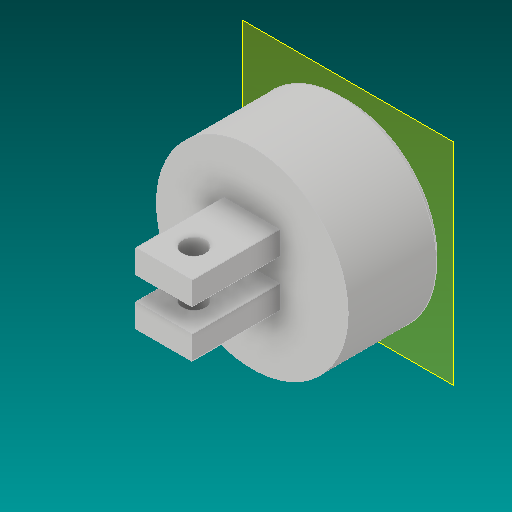
# Autodesk Inventor part: Swing_Joint_2
Saved by Autodesk Inventor 2019 (Build 230136000, 136)
## iProperties
Created: 2020-12-14
Part Number: Swing_Joint_2
Material: Generic
Document SubType Name: Modeling
Designer: Jason
Density: 1 g/cm^3
Appearance: Default
Mass: 7.35511 g
Surface Area: 26.6726 cm^2
Volume: 7.35511 cm^3
Author: Jason
Autodesk Inventor part; units mm, degrees
ref_plane "YZ Plane" through (0, 0, 0) normal (1, 0, 0) x (0, 1, 0)
ref_plane "XZ Plane" through (0, 0, 0) normal (0, 1, 0) x (-1, 0, 0)
ref_plane "XY Plane" through (0, 0, 0) normal (0, 0, 1) x (1, 0, 0)
ref_plane "Work Plane1" through (-10.8248, 8.3603, 0) normal (0, 0, 1) x (1, 0, 0)
sketch "Sketch3" plane through (-10.8248, 8.3603, 0) normal (0, 0, 1) x (1, 0, 0)
  circle A0 centre (0, 0) radius 12
  point P0 (0, 0)
  dimension "d0" = 24
  constraints: 1 centre point, 1 coincident
  measures "d0" diameter of A0
extrude "Extrusion1" add sketch "Sketch3" along normal blind 1
sketch "Sketch4" plane through (-10.8248, 8.3603, 1) normal (0, 0, 1) x (1, 0, 0)
  circle A0 centre (0, 0) radius 13
  circle A1 centre (0, 0) radius 12 projected
  dimension "d4" = 26
  constraints: 2 coincident, 1 centre point
  measures "d4" diameter of A0
extrude "Extrusion2" add sketch "Sketch4" along normal blind 12 contours A0 | A1
sketch "Sketch5" plane through (-10.8248, 8.3603, 13) normal (0, 0, 1) x (1, 0, 0)
  line L0 (-3.81, 2.1338) -> (3.81, 2.1338)
  line L1 (3.81, 2.1338) -> (3.81, 5.3088)
  line L2 (3.81, 5.3088) -> (-3.81, 5.3088)
  line L3 (-3.81, 5.3088) -> (-3.81, 2.1338)
  line L4 (-3.81, -4.2162) -> (3.81, -4.2162)
  line L5 (3.81, -4.2162) -> (3.81, -1.0412)
  line L6 (3.81, -1.0412) -> (-3.81, -1.0412)
  line L7 (-3.81, -1.0412) -> (-3.81, -4.2162)
  circle A0 centre (0, 0) radius 13 projected
  point P0 (0, -7.7939)
  dimension "d15" = 7.62
  dimension "d16" = 3.175
  dimension "d17" = 7.62
  dimension "d18" = 3.175
  dimension "d19" = 3.175
  dimension "d20" = 3.81
  dimension "d21" = 3.81
  constraints: 16 end point, 4 parallel, 2 perpendicular, 1 horizontal
  measures "d15" distance of L2.end L1.end
  measures "d16" distance of L1.end L0.end
  measures "d17" distance of L7.start L6.start
  measures "d18" distance of L6.start L4.end
  measures "d19" distance between parallel lines of L0 L6
  measures "d20" distance from line of point (0, -7.794) L1
  measures "d21" distance from line of point (0, -7.794) L5
extrude "Extrusion3" add sketch "Sketch5" along normal blind 12 contours L3 L2 L1 L0 | L7 L6 L5 L4
sketch "Sketch6" plane through (-15.5873, 4.1441, 13) normal (0, -1, 0) x (1, 0, 0)
  circle A0 centre (4.7625, 7.9375) radius 1.5685
  line L0 (0.9525, 0) -> (0.9525, 12) projected
  point P0 (4.7625, -37.7)
  dimension "d22" = 3.81
  constraints: 1 centre point
  measures "d22" distance from line of A0.centre L0
extrude "Extrusion4" cut sketch "Sketch6" against normal blind 12
body "Solid1"
